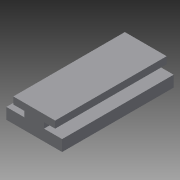
# Autodesk Inventor part: Channel I
Saved by Autodesk Inventor 2014 (Build 180170000, 170)
## iProperties
Created: 2014-07-22
Part Number: Channel I
Material: Generic
Document SubType Name: Modeling
Designer: quinn
Density: 1 g/cm^3
Appearance: Default
Author: quinn
Autodesk Inventor part; units mm, degrees
ref_plane "YZ Plane" through (0, 0, 0) normal (1, 0, 0) x (0, 1, 0)
ref_plane "XZ Plane" through (0, 0, 0) normal (0, 1, 0) x (-1, 0, 0)
ref_plane "XY Plane" through (0, 0, 0) normal (0, 0, 1) x (1, 0, 0)
sketch "Sketch1" plane through (0, 0, 0) normal (0, 0, 1) x (1, 0, 0)
  line L0 (-12.2515, 2.2665) -> (-37.6515, 2.2665)
  line L1 (-37.6515, 2.2665) -> (-37.6515, 7.3465)
  line L2 (-12.2515, 7.3465) -> (-12.2515, 2.2665)
  line L3 (-37.6515, 2.2665) -> (-12.2515, 2.2665)
  line L4 (-12.2515, 2.2665) -> (-12.2515, 7.3465)
  line L5 (-37.6515, 7.3465) -> (-37.6515, 2.2665)
  line L6 (-20.5065, 7.3465) -> (-20.5065, 9.8865)
  line L7 (-29.3965, 9.8865) -> (-29.3965, 7.3465)
  line L8 (-34.4765, 13.0615) -> (-15.4265, 13.0615)
  line L9 (-15.4265, 13.0615) -> (-15.4265, 9.8865)
  line L10 (-34.4765, 9.8865) -> (-34.4765, 13.0615)
  line L11 (-15.4265, 9.8865) -> (-20.5065, 9.8865)
  line L12 (-29.3965, 9.8865) -> (-34.4765, 9.8865)
  line L13 (-12.2515, 7.3465) -> (-20.5065, 7.3465)
  line L14 (-29.3965, 7.3465) -> (-37.6515, 7.3465)
  point P0 (0, 0)
  constraints: 30 end point, 8 parallel, 3 horizontal, 3 perpendicular
extrude "Extrusion2" add sketch "Sketch1" along normal blind 50.8
body "Solid2"
